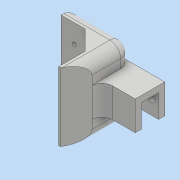
# Autodesk Inventor part: mocowanie_do_ramy
Saved by Autodesk Inventor 2017 (Build 210142000, 142)
## iProperties
Created: 2017-11-03
Part Number: mocowanie_do_ramy
Material: Ogólny
Document SubType Name: Modeling
Designer: Kuba01
Density: 1 g/cm^3
Appearance: Domyślna
Author: Kuba01
Autodesk Inventor part; units mm, degrees
ref_plane "YZ Plane" through (0, 0, 0) normal (1, 0, 0) x (0, 1, 0)
ref_plane "XZ Plane" through (0, 0, 0) normal (0, 1, 0) x (-1, 0, 0)
ref_plane "XY Plane" through (0, 0, 0) normal (0, 0, 1) x (1, 0, 0)
sketch "Szkic1" plane through (0, 0, 0) normal (0, 0, 1) x (1, 0, 0)
  point P0 (0, 0)
sketch "Szkic2" plane through (0, 0, 0) normal (0, 0, 1) x (1, 0, 0)
  line L0 (-18, 0) -> (0, 0)
  line L1 (0, 0) -> (14.4, -14.4)
  line L2 (14.4, -14.4) -> (14.4, -34.4)
  line L3 (14.4, -34.4) -> (24.4, -34.4)
  line L4 (24.4, -34.4) -> (24.4, 0)
  line L5 (24.4, 0) -> (24.4, 10)
  line L6 (24.4, 10) -> (-18, 10)
  line L7 (-18, 10) -> (-18, 0)
  dimension "d0" = 14.4
  dimension "d1" = 14.4
  dimension "d2" = 18
  dimension "d3" = 20
  dimension "d4" = 10
  dimension "d5" = 10
  constraints: 16 end point, 5 perpendicular, 1 horizontal, 1 point on line, 1 vertical
  measures "d0" horizontal distance of L1.end L0.end
  measures "d1" horizontal distance of L1.end L0.end
  measures "d2" distance from line of L7 L0.end
  measures "d3" distance from line of L3 L1.end
  measures "d4" distance between parallel lines of L6 L0
  measures "d5" distance between parallel lines of L4 L2
extrude "Wyciągnięcie proste1" add sketch "Szkic2" along normal blind 51.2
sketch "Szkic3" plane through (24.4, -34.4, 0) normal (1, 0, 0) x (0, 0, -1)
  line L0 (0, 44.4) -> (0, 0) projected
  line L1 (0, 44.4) -> (-51.2, 44.4) projected
  line L2 (-51.2, 0) -> (-51.2, 44.4) projected
  line L3 (0, 0) -> (-51.2, 0) projected
  line L4 (-36.6, 44.4) -> (-14.6, 44.4)
  line L5 (-14.6, 44.4) -> (-14.6, 22.4)
  line L6 (-14.6, 22.4) -> (-36.6, 22.4)
  line L7 (-36.6, 22.4) -> (-36.6, 44.4)
  point P0 (0, 34.4)
  point P1 (-25.6, 44.4)
  dimension "d8" = 22
  dimension "d9" = 22
  constraints: 8 end point, 2 midpoint, 2 parallel, 1 horizontal, 1 perpendicular, 1 point on line
  measures "d8" distance of L5.end L6.end
  measures "d9" distance of L4.end L5.end
extrude "Wyciągnięcie proste2" add sketch "Szkic3" along normal blind 25 contours L5 L6 L7 L1
sketch "Szkic4" plane through (49.4, -34.4, 0) normal (1, 0, 0) x (0, 0, -1)
  line L0 (-14.6, 44.4) -> (-36.6, 44.4) projected
  line L1 (-36.6, 44.4) -> (-36.6, 22.4) projected
  line L2 (-36.6, 22.4) -> (-14.6, 22.4) projected
  line L3 (-14.6, 22.4) -> (-14.6, 44.4) projected
  line L4 (-32, 39.8) -> (-19.2, 39.8)
  line L5 (-19.2, 39.8) -> (-19.2, 27)
  line L6 (-19.2, 27) -> (-32, 27)
  line L7 (-32, 27) -> (-32, 39.8)
  point P0 (0, 34.4)
  point P1 (-25.6, 39.8)
  point P2 (-25.6, 44.4)
  point P3 (-19.2, 33.4)
  point P4 (-14.6, 33.4)
  dimension "d12" = 12.8
  dimension "d13" = 12.8
  constraints: 8 end point, 4 midpoint, 2 parallel, 1 horizontal, 1 horizontal alignment, 1 perpendicular, 1 vertical alignment
  measures "d12" distance between parallel lines of L5 L7
  measures "d13" distance between parallel lines of L6 L4
extrude "Wyciągnięcie proste3" cut sketch "Szkic4" against normal blind 26 contours L4 L5 L6 L7
sketch "Szkic5" plane through (-18, 10, 0) normal (0, 1, 0) x (1, 0, 0)
  line L0 (0, 0) -> (42.4, 0) projected
  line L1 (0, 0) -> (0, -51.2) projected
  line L2 (42.4, -51.2) -> (0, -51.2) projected
  line L3 (42.4, -36.6) -> (42.4, -51.2) projected
  line L4 (42.4, -36.6) -> (67.4, -36.6) projected
  line L5 (67.4, -14.6) -> (67.4, -36.6) projected
  line L6 (42.4, -14.6) -> (67.4, -14.6) projected
  line L7 (42.4, 0) -> (42.4, -14.6) projected
  line L8 (18, 0) -> (18, -51.2) projected
  point P0 (9.9, -37.2)
  point P1 (9.9459, -23.2)
  dimension "d17" = 8.1
  dimension "d18" = 14
  dimension "d19" = 14
  measures "d17" distance from line of L8 point (9.9, -37.2)
  measures "d18" distance from line of point (9.9, -37.2) L2
  measures "d19" vertical distance of point (9.946, -23.2) point (9.9, -37.2)
hole "Otwór1" at (-8.1, 10, 37.2) at (-8.0541, 10, 23.2) direction (0, -1, 0) diameter 3 end through all
chamfer "Faza1" distance 15 angle 30 1 edges at (24.4, -34.4, 25.6) measured on face at (24.4, -26.9333, 21.9333)
fillet "Zaokrąglenie1" radius 8 1 edges at (24.4, -12, 25.6)
fillet "Zaokrąglenie2" radius 8 1 edges at (24.4, -4.7, 51.2)
fillet "Zaokrąglenie3" radius 8 1 edges at (24.4, -4.7, 0)
fillet "Zaokrąglenie4" radius 8 7 edges at (-18, 10, 25.6) (22.0569, 10, 48.8569) (24.4, 10, 39.9) (-0.8, 10, 51.2) (22.0569, 10, 2.3431) (24.4, 10, 11.3) (-0.8, 10, 0)
sketch "Szkic6" plane through (49.4, -34.4, 0) normal (1, 0, 0) x (0, 0, -1)
  line L0 (-32, 27) -> (-32, 39.8) projected
  line L1 (-32, 39.8) -> (-19.2, 39.8) projected
  line L2 (-19.2, 39.8) -> (-19.2, 27) projected
  line L3 (-19.2, 27) -> (-32, 27) projected
  line L4 (-14.6, 44.4) -> (-36.6, 44.4) projected
  line L5 (-36.6, 44.4) -> (-36.6, 22.4) projected
  line L6 (-36.6, 22.4) -> (-14.6, 22.4) projected
  line L7 (-14.6, 22.4) -> (-14.6, 44.4) projected
  line L8 (-20.5395, 39.8) -> (-13.1078, 39.8)
  line L9 (-13.1078, 39.8) -> (-13.1078, 27)
  line L10 (-13.1078, 27) -> (-20.5395, 27)
  line L11 (-20.5395, 27) -> (-20.5395, 39.8)
  point P0 (0, 34.4)
  constraints: 8 end point, 2 parallel, 1 horizontal, 1 perpendicular, 1 point on line
extrude "Wyciągnięcie proste4" cut sketch "Szkic6" against normal blind 16 contours L11 L1 L2 L3 | L2 L8 L7 L10 | L7 L8 L9 L10
sketch "Szkic7" plane through (49.4, 10, 36.6) normal (0, 1, 0) x (1, 0, 0)
  line L0 (-33, 0) -> (0, 0) projected
  line L1 (0, 22) -> (0, 0) projected
  line L2 (-33, 22) -> (0, 22) projected
  line L3 (-33, 28.6) -> (-33, 22) projected
  line L4 (-59.4, 28.6) -> (-33, 28.6) projected
  line L5 (-59.4, -6.6) -> (-59.4, 28.6) projected
  line L6 (-33, -6.6) -> (-59.4, -6.6) projected
  line L7 (-33, 0) -> (-33, -6.6) projected
  circle A0 centre (-57.5, -0.6) radius 1.5 projected
  circle A1 centre (-57.4541, 13.4) radius 1.5 projected
  point P0 (-49.4, 36.6)
  point P1 (-5, 11)
  point P2 (-20, 11)
  dimension "d36" = 5
  dimension "d37" = 15
  measures "d36" distance from line of point (-5, 11) L1
  measures "d37" distance of point (-20, 11) point (-5, 11)
hole "Otwór2" at (44.4, 10, 25.6) at (29.4, 10, 25.6) direction (0, -1, 0) diameter 5 depth 8 tip angle 118
